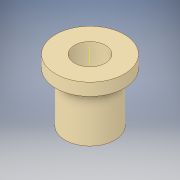
# Autodesk Inventor part: Ceramic eyelet
Saved by Autodesk Inventor 2018 (Build 220112000, 112)
## iProperties
Created: 2018-04-23
Part Number: Ceramic eyelet
Material: Generic
Document SubType Name: Modeling
Designer: pnigge
Density: 1 g/cm^3
Appearance: Exterior - Beige
Author: pnigge
Autodesk Inventor part; units mm, degrees
ref_plane "YZ Plane" through (0, 0, 0) normal (1, 0, 0) x (0, 1, 0)
ref_plane "XZ Plane" through (0, 0, 0) normal (0, 1, 0) x (-1, 0, 0)
ref_plane "XY Plane" through (0, 0, 0) normal (0, 0, 1) x (1, 0, 0)
sketch "Sketch1" plane through (0, 0, 0) normal (1, 0, 0) x (0, 1, 0)
  line L0 (-6.7792, 3.175) -> (-0.4292, 3.175)
  line L1 (-0.4292, 3.175) -> (-0.4292, 4.3815)
  line L2 (-0.4292, 4.3815) -> (1.1456, 4.3815)
  line L3 (1.1456, 4.3815) -> (1.1456, 1.9812)
  line L4 (1.1456, 1.9812) -> (-6.7792, 1.9812)
  line L5 (-6.7792, 1.9812) -> (-6.7792, 3.175)
  line L6 (-8.3642, 0) -> (2.7305, 0) projected
  point P0 (0, 0)
  dimension "d0" = 1.9812
  dimension "d1" = 3.175
  dimension "d2" = 4.3815
  dimension "d3" = 7.9248
  dimension "d4" = 6.35
  constraints: 12 end point, 4 perpendicular, 1 horizontal
  measures "d0" distance from line of point (0, 0) L4
  measures "d1" distance from line of point (0, 0) L0
  measures "d2" distance from line of point (0, 0) L2
  measures "d3" distance between parallel lines of L5 L3
  measures "d4" distance between parallel lines of L5 L1
revolve "Revolution1" add sketch "Sketch1" angle 360 about axis through (0, -10, 0) along (0, 1, 0)
body "Solid1"
